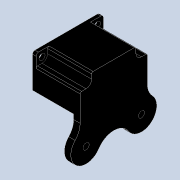
# Autodesk Inventor part: X Axis Pully Support
Saved by Autodesk Inventor 2022 (Build 260153000, 153)
## iProperties
Created: 2021-10-18
Part Number: X Axis Pully Support
Material: Generic
Document SubType Name: Modeling
Designer: Coy
Density: 1 g/cm^3
Appearance: Anodized - Black
Author: Coy
Autodesk Inventor part; units mm, degrees
ref_plane "YZ Plane" through (0, 0, 0) normal (1, 0, 0) x (0, 1, 0)
ref_plane "XZ Plane" through (0, 0, 0) normal (0, 1, 0) x (-1, 0, 0)
ref_plane "XY Plane" through (0, 0, 0) normal (0, 0, 1) x (1, 0, 0)
sketch "Sketch1" plane through (0, 0, 0) normal (1, 0, 0) x (0, 1, 0)
  arc A0 (0, -19.15) -> (0, 19.15) centre (0, 0) ccw
  line L0 (0, 28.65) -> (26.65, 28.65)
  line L1 (28.65, 26.65) -> (28.65, -26.65)
  line L2 (26.65, -28.65) -> (0, -28.65)
  line L3 (0, -28.65) -> (0, -19.15)
  line L4 (0, 19.15) -> (0, 28.65)
  arc A1 (28.65, 26.65) -> (26.65, 28.65) centre (26.65, 26.65) ccw
  arc A2 (26.65, -28.65) -> (28.65, -26.65) centre (26.65, -26.65) ccw
  line L5 (0, 23.57) -> (23.57, 23.57) construction
  line L6 (23.57, 23.57) -> (23.57, -23.57) construction
  line L7 (23.57, -23.57) -> (0, -23.57) construction
  line L8 (0, -23.57) -> (0, 23.57) construction
  circle A3 centre (23.57, 23.57) radius 2.6
  circle A4 centre (23.57, -23.57) radius 2.6
  point P0 (28.65, -28.65)
  point P1 (28.65, 28.65)
  dimension "d0" = 38.3
  dimension "d1" = 28.65
  dimension "d2" = 57.3
  dimension "d3" = 28.65
  dimension "d4" = 2
  dimension "d5" = 23.57
  dimension "d6" = 47.14
  dimension "d7" = 23.57
  dimension "d8" = 5.2
  dimension "d9" = 5.2
  constraints: 18 end point, 6 point on circle, 5 centre point, 5 parallel, 5 point on line, 4 tangent, 3 coincident, 2 horizontal, 2 perpendicular, 1 equal radius
  measures "d0" diameter of A0
  measures "d1" distance of point (28.65, -28.65) L2.end
  measures "d2" distance of point (28.65, 28.65) point (28.65, -28.65)
  measures "d3" distance from line of point (0, 0) L0
  measures "d4" radius of A1
  measures "d5" distance of L6.end L7.end
  measures "d6" distance of L5.end L6.end
  measures "d7" distance from line of point (0, 0) L5
  measures "d8" diameter of A3
  measures "d9" diameter of A4
extrude "Extrusion1" add sketch "Sketch1" along normal blind 3
sketch "Sketch2" plane through (3, 0, 0) normal (1, 0, 0) x (0, 0, -1)
  circle A0 centre (-23.57, 23.57) radius 2.6 projected
  circle A1 centre (23.57, 23.57) radius 2.6 projected
  circle A2 centre (-23.57, 23.57) radius 4.72
  circle A3 centre (23.57, 23.57) radius 4.72
  line L0 (26.65, 28.65) -> (-26.65, 28.65) projected
  line L1 (-28.65, 26.65) -> (-28.65, 0) projected
  line L2 (28.65, 0) -> (28.65, 26.65) projected
  line L3 (26.65, 28.65) -> (-26.65, 28.65) projected
  arc A4 (-26.65, 28.65) -> (-28.65, 26.65) centre (-26.65, 26.65) ccw projected
  line L4 (-28.65, 26.65) -> (-28.65, 0) projected
  line L5 (-28.65, 0) -> (-19.15, 0) projected
  arc A5 (19.15, 0) -> (-19.15, 0) centre (0, 0) ccw projected
  line L6 (19.15, 0) -> (28.65, 0) projected
  line L7 (28.65, 0) -> (28.65, 26.65) projected
  arc A6 (28.65, 26.65) -> (26.65, 28.65) centre (26.65, 26.65) ccw projected
  circle A7 centre (-23.57, 23.57) radius 2.6 projected
  circle A8 centre (23.57, 23.57) radius 2.6 projected
  line L8 (-18.85, 28.65) -> (-18.85, 23.57)
  line L9 (-28.65, 18.85) -> (-23.57, 18.85)
  line L10 (18.85, 28.65) -> (18.85, 23.57)
  line L11 (28.65, 18.85) -> (23.57, 18.85)
  arc A9 (-17.6, 28.65) -> (-18.85, 27.4) centre (-17.6, 27.4) ccw
  arc A10 (-27.4, 18.85) -> (-28.65, 17.6) centre (-27.4, 17.6) ccw
  arc A11 (18.85, 27.4) -> (17.6, 28.65) centre (17.6, 27.4) ccw
  arc A12 (28.65, 17.6) -> (27.4, 18.85) centre (27.4, 17.6) ccw
  point P0 (-2.4769, -5.2226)
  point P1 (-57.3, 46.4)
  point P2 (-57.3, 10.9)
  point P3 (0, 10.9)
  point P4 (0, 46.4)
  point P5 (-10.9124, 57.3)
  point P6 (-46.3876, 57.3)
  dimension "d34" = 2.12
  dimension "d35" = 2.12
  dimension "d36" = 2.5
  dimension "d37" = 2.5
  dimension "d38" = 2.5
  dimension "d39" = 2.5
  constraints: 12 point on circle, 12 point on line, 12 tangent, 8 end point, 6 centre point, 2 perpendicular, 2 vertical
  measures "d34" radial gap between concentric circles of A0 A2
  measures "d35" radial gap between concentric circles of A1 A3
  measures "d36" diameter of A9
  measures "d37" diameter of A10
  measures "d38" diameter of A11
  measures "d39" diameter of A12
extrude "Extrusion2" add sketch "Sketch2" along normal blind 32 contours L8 A9 L0 A11 L10 A3 L11 A12 L2 L6 A5 L5 L1 A10 L9 A2
sketch "Sketch3" plane through (35, 0, 0) normal (1, 0, 0) x (0, 0, -1)
  circle A0 centre (-23.57, 23.57) radius 2.6 construction
  line L0 (-23.57, 23.57) -> (23.57, 23.57) construction
  line L1 (23.57, 23.57) -> (23.57, -23.57) construction
  line L2 (23.57, -23.57) -> (-23.57, -23.57) construction
  line L3 (-23.57, -23.57) -> (-23.57, 23.57) construction
  circle A1 centre (-23.57, -23.57) radius 2.6
  circle A2 centre (23.57, -23.57) radius 2.6
  arc A3 (-26.65, 28.65) -> (-28.65, 26.65) centre (-26.65, 26.65) ccw projected
  line L4 (-17.6, 28.65) -> (-26.65, 28.65) projected
  line L5 (17.6, 28.65) -> (-17.6, 28.65) projected
  line L6 (26.65, 28.65) -> (17.6, 28.65) projected
  arc A4 (28.65, 26.65) -> (26.65, 28.65) centre (26.65, 26.65) ccw projected
  line L7 (0, 0) -> (-7.096, 0) construction
  arc A5 (-28.65, -26.65) -> (-26.65, -28.65) centre (-26.65, -26.65) ccw
  line L8 (-20.0479, -28.65) -> (-26.65, -28.65)
  line L9 (26.65, -28.65) -> (20.0479, -28.65)
  arc A6 (26.65, -28.65) -> (28.65, -26.65) centre (26.65, -26.65) ccw
  line L10 (-28.65, 0) -> (-19.15, 0) projected
  line L11 (19.15, 0) -> (28.65, 0) projected
  line L12 (-28.65, 0) -> (-19.15, 0) projected
  line L13 (-28.65, 0) -> (-28.65, -26.65)
  line L14 (28.65, 0) -> (28.65, 17.6) projected
  line L15 (28.65, 0) -> (28.65, -26.65)
  arc A7 (16.0392, -27.1143) -> (-16.0392, -27.1143) centre (0, -44.9767) ccw
  arc A8 (-20.0479, -28.65) -> (-16.0392, -27.1143) centre (-20.0479, -22.65) ccw
  arc A9 (16.0392, -27.1143) -> (20.0479, -28.65) centre (20.0479, -22.65) ccw
  arc A10 (19.15, 0) -> (-19.15, 0) centre (0, 0) ccw projected
  line L16 (19.15, 0) -> (28.65, 0) projected
  line L17 (28.65, 0) -> (28.65, 17.6) projected
  arc A11 (28.65, 17.6) -> (27.4, 18.85) centre (27.4, 17.6) ccw projected
  line L18 (27.4, 18.85) -> (23.57, 18.85) projected
  arc A12 (18.85, 23.57) -> (23.57, 18.85) centre (23.57, 23.57) ccw projected
  line L19 (18.85, 23.57) -> (18.85, 27.4) projected
  arc A13 (18.85, 27.4) -> (17.6, 28.65) centre (17.6, 27.4) ccw projected
  line L20 (17.6, 28.65) -> (-17.6, 28.65) projected
  arc A14 (-17.6, 28.65) -> (-18.85, 27.4) centre (-17.6, 27.4) ccw projected
  line L21 (-18.85, 27.4) -> (-18.85, 23.57) projected
  arc A15 (-23.57, 18.85) -> (-18.85, 23.57) centre (-23.57, 23.57) ccw projected
  line L22 (-23.57, 18.85) -> (-27.4, 18.85) projected
  arc A16 (-27.4, 18.85) -> (-28.65, 17.6) centre (-27.4, 17.6) ccw projected
  line L23 (-28.65, 17.6) -> (-28.65, 0) projected
  line L24 (-28.65, 0) -> (-19.15, 0) projected
  circle A17 centre (23.57, -23.57) radius 13
  circle A18 centre (-23.57, -23.57) radius 13
  point P0 (-17.6, -28.65)
  point P1 (17.6, -28.65)
  point P2 (10.5708, -23.4226)
  point P3 (28.65, -11.6036)
  point P4 (-28.65, -11.6036)
  point P5 (-10.5708, -23.4226)
  dimension "d42" = 47.14
  dimension "d43" = 47.14
  dimension "d44" = 5.2
  dimension "d45" = 5.2
  dimension "d46" = 6
  dimension "d49" = 26
  dimension "d50" = 26
  constraints: 18 end point, 12 point on circle, 9 centre point, 8 symmetric about line, 5 tangent, 4 coincident, 3 parallel, 2 horizontal, 2 point on line, 1 collinear, 1 equal radius, 1 perpendicular, 2 other
  measures "d42" distance of L1.end L2.end
  measures "d43" distance of L0.end L1.end
  measures "d44" diameter of A1
  measures "d45" diameter of A2
  measures "d46" radius of A8
  measures "d49" diameter of A17
  measures "d50" diameter of A18
extrude "Extrusion3" add sketch "Sketch3" along normal blind 5.5
fillet "Fillet1" radius 15 4 edges at (37.75, -11.6036, 28.65) (37.75, -11.6036, -28.65) (37.75, -23.4226, 10.5708) (37.75, -23.4226, -10.5708)
equation "\"d3\" = 0.5 * d2"
equation "\"d7\" = d5"
equation "\"d9\" = d8"
equation "\"d37\" = d36"
equation "\"d38\" = d36"
equation "\"d39\" = d36"
body "Solid1"
